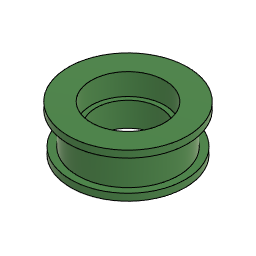
PicoPlotter (Autodesk Fusion 360 archive; units mm, degrees)
design "pulley"
Autodesk Fusion 360 part; units mm, degrees
sketch "Sketch3" plane through (0, 0, 0) normal (0, 0, 1) x (1, 0, 0)
  circle A0 centre (26.3947, 0) radius 8
  circle A1 centre (26.3947, 0) radius 11
  dimension "d13" = 16
  dimension "d14" = 22
  constraint concentric A0 A1
  measures "d13" diameter of A0
  measures "d14" diameter of A1
extrude "Extrude4" add sketch "Sketch3" along normal blind 10
sketch "Sketch4" plane through (0, 0, 10) normal (0, 0, 1) x (-1, 0, 0)
  circle A0 centre (-26.3947, 0) radius 8
  circle A1 centre (-26.3947, 0) radius 11
  circle A2 centre (-26.3947, 0) radius 13
  circle A3 centre (-26.3947, 0) radius 8
  dimension "d17" = 26
  constraint concentric A2 A3
  measures "d17" diameter of A2
extrude "Extrude5" add sketch "Sketch4" against normal blind 1.5 contours A2
sketch "Sketch5" plane through (0, 0, 0) normal (0, 0, -1) x (1, 0, 0)
  circle A0 centre (26.3947, 0) radius 8
  circle A1 centre (26.3947, 0) radius 11
  circle A2 centre (26.3947, 0) radius 12.5
  dimension "d20" = 25
  constraint concentric A0 A2
  measures "d20" diameter of A2
extrude "Extrude6" add sketch "Sketch5" against normal blind 1.5 contours A2
fillet "Fillet2" radius 1 1 edges at (16.1391, 3.9778, 8.5)
sketch "Sketch6" plane through (0, 0, 0) normal (0, 0, -1) x (1, 0, 0)
  circle A0 centre (26.3947, 0) radius 12.5
  circle A1 centre (26.3947, 0) radius 8
  circle A2 centre (26.3947, 0) radius 7
  dimension "d25" = 14
  constraint concentric A0 A2
  measures "d25" diameter of A2
extrude "Extrude7" add sketch "Sketch6" against normal blind 5.3 contours A1
